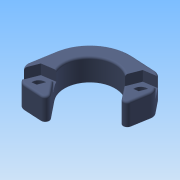
# Autodesk Inventor part: крпеление хотэнда e3dv6
Saved by Autodesk Inventor 2017 (Build 210142000, 142)
## iProperties
Part Number: крпеление хотэнда e3dv6
Material: Типовые
Document SubType Name: Modeling
Designer: Max
Mass: 0.830465 g
Surface Area: 9.06937 cm^2
Volume: 0.830465 cm^3
Density: 1 g/cm^3
Appearance: Резина — синяя
Author: Max
Autodesk Inventor part; units mm, degrees
ref_plane "YZ Plane" through (0, 0, 0) normal (1, 0, 0) x (0, 1, 0)
ref_plane "XZ Plane" through (0, 0, 0) normal (0, 1, 0) x (-1, 0, 0)
ref_plane "XY Plane" through (0, 0, 0) normal (0, 0, 1) x (1, 0, 0)
sketch "Эскиз1" plane through (0, 0, 0) normal (0, 0, 1) x (1, 0, 0)
  circle A0 centre (8, 0) radius 6 construction
  circle A1 centre (0.968872, -5.618118) radius 2.517691 construction
  circle A2 centre (15.031128, 5.618118) radius 2.517691 construction
  arc A3 (12.804604, 3.839047) -> (3.195396, -3.839047) centre (8, 0) ccw
  circle A4 centre (0.968872, -5.618118) radius 1.65
  circle A5 centre (15.031128, 5.618118) radius 1.65
  line L0 (8, 0) -> (0.968872, -5.618118) construction
  line L1 (8, 0) -> (17.430138, -11.801907) construction
  line L2 (3.195396, -3.839047) -> (8.136643, -10.023065)
  line L3 (12.804604, 3.839047) -> (17.745851, -2.344971)
  line L4 (-2.975535, -4.953548) -> (-1.861018, 1.661424)
  line L5 (0.746685, -9.611942) -> (8.136643, -10.023065)
  line L6 (18.975535, 4.953548) -> (17.745851, -2.344971)
  line L7 (8.555467, 9.984561) -> (15.253315, 9.611942)
  arc A6 (8.555467, 9.984561) -> (-1.861018, 1.661424) centre (8, 0) ccw
  arc A7 (2.007079, 0.291377) -> (1.858104, 0.315622) centre (0.968872, -5.618118) ccw
  arc A8 (-2.975535, -4.953548) -> (0.746685, -9.611942) centre (0.968872, -5.618118) ccw
  arc A9 (6.944334, -6.160201) -> (6.961793, -5.909495) centre (0.968872, -5.618118) ccw
  arc A10 (13.992921, -0.291377) -> (14.241299, -0.32967) centre (15.031128, 5.618118) ccw
  arc A11 (18.975535, 4.953548) -> (15.253315, 9.611942) centre (15.031128, 5.618118) ccw
  arc A12 (9.047432, 6.060147) -> (9.038207, 5.909495) centre (15.031128, 5.618118) ccw
  point P0 (0, 0)
  dimension "d0" = 12.3
  dimension "d1" = 3.3
  dimension "d2" = 3.3
  dimension "d3" = 90
  dimension "d7" = 10
  dimension "d8" = 4
  dimension "d9" = 4
  constraints: 22 point on circle, 16 end point, 10 centre point, 8 tangent, 6 coincident, 2 perpendicular, 1 point on line, 2 other
  measures "d0" diameter of A3
  measures "d1" diameter of A4
  measures "d2" diameter of A5
  measures "d3" angle of L1 L0
  measures "d7" radius of A6
  measures "d8" radius of A8
  measures "d9" radius of A11
extrude "Выдавливание1" add sketch "Эскиз1" along normal blind 5.9
sketch "Эскиз3" plane through (0, 0, 5.9) normal (0, 0, 1) x (1, 0, 0)
  circle A0 centre (15.031128, 5.618118) radius 1.65
  circle A1 centre (0.968872, -5.618118) radius 1.65
  arc A2 (12.804604, 3.839047) -> (3.195396, -3.839047) centre (8, 0) ccw
  line L0 (12.804604, 3.839047) -> (17.745851, -2.344971)
  line L1 (17.745851, -2.344971) -> (18.975535, 4.953548)
  arc A3 (18.975535, 4.953548) -> (15.253315, 9.611942) centre (15.031128, 5.618118) ccw
  line L2 (15.253315, 9.611942) -> (8.555467, 9.984561)
  arc A4 (8.555467, 9.984561) -> (-1.861018, 1.661424) centre (8, 0) ccw
  line L3 (-1.861018, 1.661424) -> (-2.975535, -4.953548)
  arc A5 (-2.975535, -4.953548) -> (0.746685, -9.611942) centre (0.968872, -5.618118) ccw
  line L4 (0.746685, -9.611942) -> (8.136643, -10.023065)
  line L5 (8.136643, -10.023065) -> (3.195396, -3.839047)
  line L6 (0.968872, -5.618118) -> (15.031128, 5.618118) construction
  line L7 (-1.049381, -3.092254) -> (2.147208, -2.607327)
  line L8 (2.147208, -2.607327) -> (4.165461, -5.133191)
  line L9 (4.165461, -5.133191) -> (2.987126, -8.143981)
  line L10 (2.987126, -8.143981) -> (-0.209463, -8.628908)
  line L11 (-0.209463, -8.628908) -> (-2.227716, -6.103045)
  line L12 (-2.227716, -6.103045) -> (-1.049381, -3.092254)
  line L13 (13.012874, 8.143981) -> (16.209463, 8.628908)
  line L14 (16.209463, 8.628908) -> (18.227716, 6.103045)
  line L15 (18.227716, 6.103045) -> (17.049381, 3.092254)
  line L16 (17.049381, 3.092254) -> (13.852792, 2.607327)
  line L17 (13.852792, 2.607327) -> (11.834539, 5.133191)
  line L18 (11.775027, 4.981131) -> (13.012874, 8.143981)
  line L19 (2.147208, -2.607327) -> (2.308651, -2.582836)
  arc A6 (12.804604, 3.839047) -> (3.195396, -3.839047) centre (8, 0) ccw
  arc A7 (2.308651, -2.582836) -> (2.663821, -3.253874) centre (8, 0) ccw
  arc A8 (12.351152, 4.486644) -> (11.775027, 4.981131) centre (8, 0) ccw
  point P0 (0, 0)
  dimension "d12" = 5.6
  dimension "d13" = 5.6
  constraints: 28 end point, 4 point on circle, 3 point on line, 2 centre point, 2 coincident, 2 perpendicular, 1 collinear, 33 other
  measures "d12" distance between parallel lines of L11 L8
  measures "d13" distance between parallel lines of L14 L17
extrude "Выдавливание2" cut sketch "Эскиз3" against normal blind 2.5 contours L7 L8 L9 L10 L11 L12 | L19 A7 L8 | L13 L14 L15 L16 L17 L18 | L17 A8 L18
fillet "Сопряжение1" radius 1 2 edges at (8.1366, -10.0231, 2.95) (17.7459, -2.345, 2.95)
sketch "Эскиз4" plane through (0, 0, 5.9) normal (0, 0, 1) x (1, 0, 0)
  line L0 (17.049381, 3.092254) -> (13.852792, 2.607327)
  line L1 (18.227716, 6.103045) -> (17.049381, 3.092254)
  line L2 (16.209463, 8.628908) -> (18.227716, 6.103045)
  line L3 (13.012874, 8.143981) -> (16.209463, 8.628908)
  line L4 (11.775027, 4.981131) -> (13.012874, 8.143981)
  circle A0 centre (15.031128, 5.618118) radius 1.65
  line L5 (-1.049381, -3.092254) -> (2.308651, -2.582836)
  line L6 (-2.227716, -6.103045) -> (-1.049381, -3.092254)
  line L7 (-0.209463, -8.628908) -> (-2.227716, -6.103045)
  line L8 (2.987126, -8.143981) -> (-0.209463, -8.628908)
  line L9 (4.165461, -5.133191) -> (2.987126, -8.143981)
  circle A1 centre (0.968872, -5.618118) radius 1.65
  line L10 (12.882727, 12.792349) -> (20.347901, 3.449613)
  line L11 (20.347901, 3.449613) -> (20.190459, 12.113666)
  line L12 (20.190459, 12.113666) -> (13.381128, 14.32622)
  line L13 (13.381128, 14.32622) -> (12.882727, 12.792349)
  line L14 (-4.209929, -3.622286) -> (2.790028, -12.382799)
  line L15 (2.790028, -12.382799) -> (-2.227716, -19.3644)
  line L16 (-2.227716, -19.3644) -> (-8.07565, -12.045656)
  arc A2 (-8.07565, -10.247273) -> (-8.07565, -12.045656) centre (-6.950304, -11.146464) ccw
  line L17 (-8.07565, -10.247273) -> (-8.650245, -1.51949)
  line L18 (-8.650245, -1.51949) -> (-8.07565, -1.481661)
  line L19 (-8.07565, -1.481661) -> (-4.209929, -3.622286)
  line L20 (2.663821, -3.253874) -> (4.165461, -5.133191)
  arc A3 (2.308651, -2.582836) -> (2.663821, -3.253874) centre (8, 0) ccw
  arc A4 (12.351152, 4.486644) -> (11.775027, 4.981131) centre (8, 0) ccw
  line L21 (13.852792, 2.607327) -> (12.351152, 4.486644)
  point P0 (0, 0)
  constraints: 20 end point, 2 parallel, 2 point on circle, 1 centre point, 1 perpendicular, 1 tangent
extrude "Выдавливание3" cut sketch "Эскиз4" against normal blind 10 contours L2 L10 L13 L12 L11 | L7 L14 L15 L16 A2 L17 L18 L19
fillet "Сопряжение3" radius 2 4 edges at (0.5646, -9.5976, 2.95) (-3.0018, -5.1343, 2.95) (15.4354, 9.5976, 2.95) (19.0018, 5.1343, 2.95)
fillet "Сопряжение4" radius 0.5 18 edges at (6.8484, -9.3587, 5.9) (4.9681, -6.0576, 5.9) (0.6556, -9.4323, 5.9) (-0.0999, -8.7661, 5.9) (3.6826, -9.7753, 5.9) (-2.3588, -1.2933, 5.9) (-2.8205, -5.0821, 5.9) (-2.3373, -5.9659, 5.9) (11.5472, 9.8181, 5.9) (15.3444, 9.4323, 5.9) (16.0999, 8.7661, 5.9) (1.7576, 7.8124, 5.9) (18.8205, 5.0821, 5.9) (18.3373, 5.9659, 5.9) (17.3822, -0.9418, 5.9) (14.5773, 1.6205, 5.9) (18.487, 2.054, 5.9) (4.161, 4.8046, 5.9)
sketch "Эскиз5" plane through (0, 0, 5.9) normal (0, 0, 1) x (1, 0, 0)
  circle A0 centre (0.968872, -5.618118) radius 1.65
  line L0 (-1.049381, -3.092254) -> (2.308651, -2.582836)
  line L1 (-2.227716, -6.103045) -> (-1.049381, -3.092254)
  line L2 (-0.209463, -8.628908) -> (-2.227716, -6.103045)
  line L3 (2.987126, -8.143981) -> (-0.209463, -8.628908)
  line L4 (4.165461, -5.133191) -> (2.987126, -8.143981)
  line L5 (2.663821, -3.253874) -> (4.165461, -5.133191)
  arc A1 (2.308651, -2.582836) -> (2.663821, -3.253874) centre (8, 0) ccw
  circle A2 centre (15.031128, 5.618118) radius 1.65
  line L6 (13.012874, 8.143981) -> (16.209463, 8.628908)
  line L7 (11.775027, 4.981131) -> (13.012874, 8.143981)
  arc A3 (12.351152, 4.486644) -> (11.775027, 4.981131) centre (8, 0) ccw
  line L8 (13.852792, 2.607327) -> (12.351152, 4.486644)
  line L9 (17.049381, 3.092254) -> (13.852792, 2.607327)
  line L10 (18.227716, 6.103045) -> (17.049381, 3.092254)
  line L11 (16.209463, 8.628908) -> (18.227716, 6.103045)
  line L12 (11.775027, 4.981131) -> (2.308651, -2.582836)
  line L13 (4.165461, -5.133191) -> (2.987126, -8.143981)
  line L14 (4.165461, -5.133191) -> (13.852792, 2.607327)
  point P0 (0, 0)
  constraints: 4 end point, 1 parallel
extrude "Выдавливание4" cut sketch "Эскиз5" against normal up to surface (2.5 mm away) contours A0 | L0 A1 L5 L4 L3 L2 L1 | L12 A3 L8 L14 L5 A1 | L7 L6 L11 L10 L9 L8 A3 | A2
